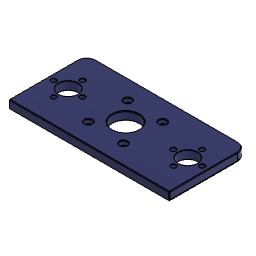
Motor Bracket v4 (Autodesk Fusion 360 design; units mm, degrees)
Autodesk Fusion 360 part; units mm, degrees
sketch "Sketch2" plane through (0, 0, 0) normal (0, 0, 1) x (1, 0, 0)
  line L0 (0, 0) -> (134, 0)
  line L1 (134, 0) -> (134, 57)
  line L2 (126, 65) -> (8, 65)
  line L3 (0, 57) -> (0, 0)
  circle A0 centre (64.9939, 32.5034) radius 11
  circle A1 centre (17, 32.5) radius 4
  circle A2 centre (117, 32.5) radius 4
  circle A3 centre (50.3426, 48.915) radius 1.5
  circle A4 centre (80.5569, 48.0531) radius 1.5
  circle A5 centre (49.4456, 16.939) radius 1.5
  circle A6 centre (79.6451, 16.0918) radius 1.5
  arc A7 (8, 65) -> (0, 57) centre (8, 57) ccw
  arc A8 (134, 57) -> (126, 65) centre (126, 57) ccw
  point P0 (0, 65)
  dimension "d1" = 134
  dimension "d2" = 65
  dimension "d6" = 8
  dimension "d8" = 8
  dimension "d32" = 3
  dimension "d34" = 3
  dimension "d36" = 3
  dimension "d38" = 3
  dimension "d39" = 8
  dimension "d40" = 8
  constraint horizontal L0
  constraint vertical L1
  constraint horizontal L2
  constraint vertical L3
  constraint coincident L0.start L3.end
  constraint coincident P0 L2
  constraint coincident P0 L3
  constraint tangent L2 A7
  constraint tangent L3 A7
  constraint tangent L1 A8
  constraint tangent L2 A8
  measures "d1" distance of L0.start L0.end
  measures "d2" distance of L0.start P0
  measures "d6" diameter of A1
  measures "d8" diameter of A2
  measures "d32" diameter of A3
  measures "d34" diameter of A4
  measures "d36" diameter of A5
  measures "d38" diameter of A6
  measures "d39" radius of A7
  measures "d40" radius of A8
extrude "Extrude1" add sketch "Sketch2" along normal blind 7 makes body 1
sketch "Sketch3" plane through (0, 0, 7) normal (0, 0, 1) x (-1, 0, 0)
  circle A0 centre (-17, -32.5) radius 4
  circle A1 centre (-64.9939, -32.5034) radius 11
  circle A2 centre (-50.3426, -48.915) radius 1.5
  circle A3 centre (-80.5569, -48.0531) radius 1.5
  circle A4 centre (-117, -32.5) radius 4
  circle A5 centre (-79.6451, -16.0918) radius 1.5
  circle A6 centre (-49.4456, -16.939) radius 1.5
  arc A7 (-134, -57) -> (-126, -65) centre (-126, -57) ccw
  line L0 (-126, -65) -> (-8, -65)
  arc A8 (-8, -65) -> (0, -57) centre (-8, -57) ccw
  line L1 (0, -57) -> (0, 0)
  line L2 (0, 0) -> (-134, 0)
  line L3 (-134, 0) -> (-134, -57)
  circle A9 centre (-50.3426, -48.915) radius 3
  circle A10 centre (-80.5569, -48.0531) radius 3
  circle A11 centre (-79.6451, -16.0918) radius 3
  circle A12 centre (-49.4456, -16.939) radius 3
  dimension "d43" = 6
  dimension "d44" = 6
  dimension "d45" = 6
  dimension "d46" = 6
  constraint concentric A2 A9
  constraint concentric A3 A10
  constraint concentric A5 A11
  constraint concentric A6 A12
  measures "d43" diameter of A9
  measures "d44" diameter of A10
  measures "d45" diameter of A11
  measures "d46" diameter of A12
extrude "Extrude2" cut sketch "Sketch3" against normal blind 3.5 contours A9 | A10 | A11 | A12 bodies 1
copy_body "Body->Comp1" bodies 1 removing the originals makes body 2 in component "Motor Bracket"
chamfer "Chamfer1" distance 0.5 angle 45 1 edges at (13.2707, 33.9465, 7) on bodies 2 in component "Motor Bracket"
chamfer "Chamfer2" distance 0.5 angle 45 1 edges at (53.1396, 47.8301, 7) on bodies 2 in component "Motor Bracket"
chamfer "Chamfer3" distance 0.5 angle 45 6 edges at (83.3539, 46.9682, 7) (52.2426, 15.8541, 7) (61.0161, 22.2478, 7) (82.4421, 15.007, 7) (67, 0, 7) (113.2707, 33.9465, 7) on bodies 2 in component "Motor Bracket"
chamfer "Chamfer4" distance 0.2 angle 45 1 edges at (79.1584, 47.5107, 3.5) on bodies 2 in component "Motor Bracket"
chamfer "Chamfer5" distance 0.2 angle 45 1 edges at (48.9441, 48.3726, 3.5) on bodies 2 in component "Motor Bracket"
chamfer "Chamfer6" distance 0.2 angle 45 1 edges at (48.0471, 16.3965, 3.5) on bodies 2 in component "Motor Bracket"
chamfer "Chamfer7" distance 0.2 angle 45 1 edges at (78.2467, 15.5494, 3.5) on bodies 2 in component "Motor Bracket"
chamfer "Chamfer8" distance 0.5 angle 45 1 edges at (13.2707, 33.9465, 0) on bodies 2 in component "Motor Bracket"
chamfer "Chamfer9" distance 0.5 angle 45 6 edges at (48.0471, 17.4814, 0) (48.9441, 49.4574, 0) (61.0161, 22.2478, 0) (79.1584, 48.5955, 0) (78.2467, 16.6342, 0) (113.2707, 33.9465, 0) on bodies 2 in component "Motor Bracket"
chamfer "Chamfer10" distance 0.5 angle 45 1 edges at (67, 0, 0) on bodies 2 in component "Motor Bracket"
chamfer "Chamfer11" distance 0.5 angle 45 5 edges at (134, 28.75, 0) (131.6569, 62.6569, 0) (67, 65, 0) (2.3431, 62.6569, 0) (0, 28.75, 0) on bodies 2 in component "Motor Bracket"
chamfer "Chamfer12" distance 0.5 angle 45 5 faces at (0, 19.1667, 2.6667) (1.4834, 61.6405, 4.8333) (86.6667, 65, 2.6667) (126.3807, 64.9909, 4.8333) (134, 19.1667, 2.6667) on bodies 2 in component "Motor Bracket"
sketch "Sketch4" plane through (0, 0, 7) normal (0, 0, 1) x (-1, 0, 0)
  line L0 (-0.5, -57) -> (-0.5, -0.5)
  line L1 (-0.5, -0.5) -> (-133.5, -0.5)
  line L2 (-133.5, -0.5) -> (-133.5, -57)
  arc A0 (-133.5, -57) -> (-126, -64.5) centre (-126, -57) ccw
  line L3 (-126, -64.5) -> (-8, -64.5)
  arc A1 (-8, -64.5) -> (-0.5, -57) centre (-8, -57) ccw
  circle A2 centre (-64.9939, -32.5034) radius 11.5
  circle A3 centre (-80.5569, -48.0531) radius 3.5
  circle A4 centre (-17, -32.5) radius 4.5
  circle A5 centre (-50.3426, -48.915) radius 3.5
  circle A6 centre (-49.4456, -16.939) radius 3.5
  circle A7 centre (-79.6451, -16.0918) radius 3.5
  circle A8 centre (-117, -32.5) radius 4.5
  circle A9 centre (-17, -32.5) radius 8
  line L4 (-17, -32.5) -> (-17, -44.5)
  line L5 (-17, -32.5) -> (-17, -20.5)
  line L6 (-17, -32.5) -> (-29, -32.5)
  line L7 (-17, -32.5) -> (-5, -32.5)
  circle A10 centre (-17, -44.5) radius 2
  circle A11 centre (-29, -32.5) radius 2
  circle A12 centre (-17, -20.5) radius 2
  circle A13 centre (-5, -32.5) radius 2
  circle A14 centre (-117, -32.5) radius 8
  line L8 (-117, -32.5) -> (-117, -44.5)
  line L9 (-117, -32.5) -> (-129, -32.5)
  line L10 (-117, -32.5) -> (-105, -32.5)
  line L11 (-117, -32.5) -> (-117, -20.5)
  circle A15 centre (-117, -44.5) radius 2
  circle A16 centre (-129, -32.5) radius 2
  circle A17 centre (-117, -20.5) radius 2
  circle A18 centre (-105, -32.5) radius 2
  dimension "d61" = 16
  dimension "d62" = 12
  dimension "d63" = 12
  dimension "d64" = 12
  dimension "d65" = 12
  dimension "d66" = 4
  dimension "d67" = 4
  dimension "d68" = 4
  dimension "d69" = 4
  dimension "d70" = 16
  dimension "d71" = 12
  dimension "d72" = 12
  dimension "d73" = 12
  dimension "d74" = 12
  dimension "d75" = 4
  dimension "d76" = 4
  dimension "d77" = 4
  dimension "d78" = 4
  constraint concentric A4 A9
  constraint coincident A4.centre A9.centre
  constraint vertical L4
  constraint parallel L4 L5
  constraint perpendicular L4 L6
  constraint perpendicular L4 L7
  constraint coincident L4.end A10.centre
  constraint coincident L6.end A11.centre
  constraint coincident L5.end A12.centre
  constraint coincident L7.end A13.centre
  constraint concentric A8 A14
  constraint coincident A8.centre A14.centre
  constraint vertical L8
  constraint perpendicular L8 L9
  constraint perpendicular L8 L10
  constraint perpendicular L9 L11
  constraint coincident L8.end A15.centre
  constraint coincident L9.end A16.centre
  constraint coincident L11.end A17.centre
  constraint coincident L10.end A18.centre
  measures "d61" diameter of A9
  measures "d62" distance of A4.centre L4.end
  measures "d63" distance of A4.centre L5.end
  measures "d64" distance of A4.centre L6.end
  measures "d65" distance of A4.centre L7.end
  measures "d66" diameter of A10
  measures "d67" diameter of A11
  measures "d68" diameter of A12
  measures "d69" diameter of A13
  measures "d70" diameter of A14
  measures "d71" distance of A8.centre L8.end
  measures "d72" distance of A8.centre L9.end
  measures "d73" distance of A8.centre L10.end
  measures "d74" distance of A8.centre L11.end
  measures "d75" diameter of A15
  measures "d76" diameter of A16
  measures "d77" diameter of A17
  measures "d78" diameter of A18
extrude "Extrude1'" cut sketch "Sketch4" against normal blind 30 contours A4 L5 L7 | A4 A9 L4 L7 | A4 L4 L7 | A4 A9 L5 L7 | A4 L5 L6 | A4 A9 L5 L6 | A4 A9 L4 L6 | A4 L4 L6 | A8 L10 L11 | A8 A14 L8 L10 | A8 L8 L10 | A8 A14 L10 L11 | A8 L9 L11 | A8 A14 L9 L11 | A8 A14 L8 L9 | A8 L8 L9 | A10 | A11 | A12 | A13 | A15 | A16 | A17 | A18 bodies 2 in component "Motor Bracket"
chamfer "Chamfer13" distance 0.2 angle 45 10 edges at (6.8647, 31.7768, 7) (18.8647, 43.7768, 7) (30.8647, 31.7768, 7) (24.4586, 29.6071, 7) (18.8647, 19.7768, 7) (124.4586, 29.6071, 7) (118.8647, 43.7768, 7) (106.8647, 31.7768, 7) (118.8647, 19.7768, 7) (130.8647, 31.7768, 7) on bodies 2 in component "Motor Bracket"
chamfer "Chamfer14" distance 0.2 angle 45 10 edges at (118.8647, 45.2232, 0) (124.4586, 35.3929, 0) (130.8647, 33.2232, 0) (118.8647, 21.2232, 0) (106.8647, 33.2232, 0) (30.8647, 33.2232, 0) (18.8647, 45.2232, 0) (6.8647, 33.2232, 0) (18.8647, 21.2232, 0) (24.4586, 35.3929, 0) on bodies 2 in component "Motor Bracket"
component "Motor Bracket" placed x (1, 0, 0) y (0, 1, 0) z (0, 0, 1) at (0, 0, 0)
